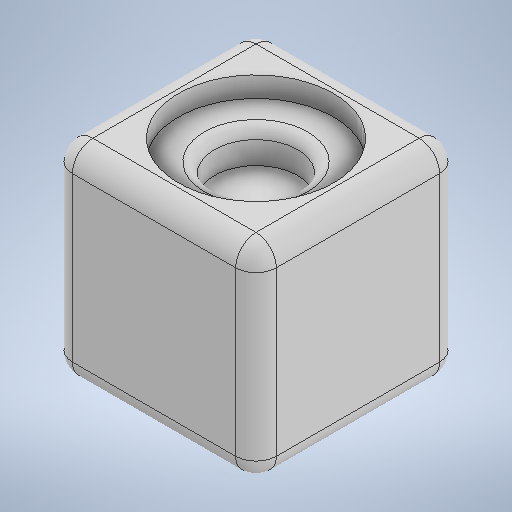
# Autodesk Inventor part: Center
Saved by Autodesk Inventor 2025 (Build 290162000, 162)
## iProperties
Created: 2026-02-12
Part Number: Center
Material: Generic
Document SubType Name: Modeling
Designer: tapen
Density: 1 g/cm^3
Appearance: Default
Author: tapen
Autodesk Inventor part; units mm, degrees
ref_plane "YZ Plane" through (0, 0, 0) normal (1, 0, 0) x (0, 1, 0)
ref_plane "XZ Plane" through (0, 0, 0) normal (0, 1, 0) x (-1, 0, 0)
ref_plane "XY Plane" through (0, 0, 0) normal (0, 0, 1) x (1, 0, 0)
sketch "Sketch1" plane through (0, 0, 0) normal (0, 0, 1) x (1, 0, 0)
  line L0 (-10, -10) -> (10, -10)
  line L1 (10, -10) -> (10, 10)
  line L2 (10, 10) -> (-10, 10)
  line L3 (-10, 10) -> (-10, -10)
  line L4 (-10, -10) -> (10, 10) construction
  line L5 (10, -10) -> (-10, 10) construction
  point P0 (0, 0)
  dimension "d0" = 20
  dimension "d1" = 20
  constraints: 12 end point, 2 midpoint, 2 parallel, 1 horizontal, 1 perpendicular
  measures "d0" distance of L2.end L1.end
  measures "d1" distance of L1.end L0.end
extrude "Extrusion1" add sketch "Sketch1" along normal blind 20
sketch "Sketch2" plane through (-10, 10, 0) normal (0, 1, 0) x (1, 0, 0)
  circle A0 centre (10, -10) radius 7.6
  line L0 (0, 0) -> (0, -20) projected
  point P0 (10, 0)
  dimension "d4" = 15.2
  dimension "d5" = 10
  dimension "d6" = 10
  constraints: 1 centre point
  measures "d4" diameter of A0
  measures "d5" distance of point (10, 0) A0.centre
  measures "d6" distance from line of L0 A0.centre
extrude "Extrusion2" cut sketch "Sketch2" against normal blind 2
sketch "Sketch3" plane through (0, 0, 0) normal (0, 0, -1) x (-1, 0, 0)
  circle A0 centre (0, 0) radius 7.6
  dimension "d9" = 15.2
  constraints: 1 centre point, 1 coincident
  measures "d9" diameter of A0
extrude "Extrusion3" cut sketch "Sketch3" against normal blind 2
sketch "Sketch4" plane through (-10, -10, 0) normal (-1, 0, 0) x (0, 0, 1)
  circle A0 centre (10, 10) radius 7.6
  line L0 (0, 20) -> (0, 0) projected
  line L1 (0, 20) -> (20, 20) projected
  point P0 (0, 10)
  dimension "d12" = 15.2
  dimension "d13" = 10
  dimension "d14" = 10
  constraints: 1 centre point
  measures "d12" diameter of A0
  measures "d13" distance from line of L0 A0.centre
  measures "d14" distance from line of L1 A0.centre
extrude "Extrusion4" cut sketch "Sketch4" against normal blind 2
fillet "Fillet1" radius 2 11 edges at (-10, 10, 10) (0, 10, 20) (-10, 0, 20) (-10, 0, 0) (0, -10, 0) (10, 0, 0) (0, 10, 0) (10, 10, 10) (10, -10, 10) (0, -10, 20) (10, 0, 20)
sketch "Sketch5" plane through (-8, 0, 10) normal (-1, 0, 0) x (0, 0, 1)
  circle A0 centre (0, 0) radius 4.07
  point P0 (-10, 0)
  dimension "d18" = 8.14
  constraints: 1 centre point
  measures "d18" diameter of A0
extrude "Extrusion5" cut sketch "Sketch5" against normal blind 3.2
sketch "Sketch6" plane through (0, 0, 2) normal (0, 0, -1) x (-1, 0, 0)
  circle A0 centre (0, 0) radius 3.98
  dimension "d21" = 7.96
  constraints: 1 centre point, 1 coincident
  measures "d21" diameter of A0
extrude "Extrusion6" cut sketch "Sketch6" against normal blind 3.2
sketch "Sketch7" plane through (0, 8, 10) normal (0, 1, 0) x (1, 0, 0)
  circle A0 centre (0, 0) radius 4.07
  point P0 (0, 10)
  dimension "d24" = 8.14
  constraints: 1 centre point
  measures "d24" diameter of A0
extrude "Extrusion7" cut sketch "Sketch7" against normal blind 3.2
fillet "Fillet2" radius 2 3 edges at (-9.4142, -9.4142, 19.4142) (-9.4142, -9.4142, 0.5858) (-10, -10, 10)
fillet "Fillet3" radius 1 1 edges at (-8, 0, 5.93)
fillet "Fillet4" radius 1 1 edges at (-4.07, 8, 10)
fillet "Fillet5" radius 1 1 edges at (3.98, 0, 2)
equation "\"d1\" = d0"
equation "\"d6\" = d5"
equation "\"d13\" = d14"
body "Solid1"
